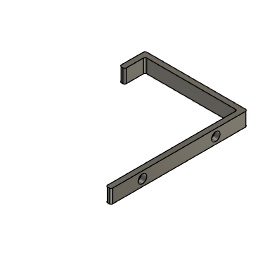
Dell Monitor Mount (Autodesk Fusion 360 design; units mm, degrees)
Autodesk Fusion 360 part; units mm, degrees
sketch "Sketch1" plane through (0, 0, 0) normal (0, 0, 1) x (1, 0, 0)
  line L0 (0, 0) -> (3, 0)
  line L1 (3, 0) -> (3, 80)
  line L2 (3, 80) -> (0, 80)
  line L3 (0, 77) -> (0, 0)
  line L4 (0, 80) -> (-57, 80)
  line L5 (-57, 80) -> (-57, 77)
  line L6 (-54, 77) -> (0, 77)
  line L7 (-54, 77) -> (-54, 65)
  line L8 (-54, 65) -> (-57, 65)
  line L9 (-57, 65) -> (-57, 77)
  dimension "d1" = 80
  dimension "d2" = 3
  dimension "d3" = 60
  dimension "d4" = 3
  dimension "d5" = 15
  dimension "d6" = 3
  constraint horizontal L0
  constraint vertical L1
  constraint horizontal L2
  constraint vertical L3
  constraint coincident L0.start L3.end
  constraint horizontal L4
  constraint vertical L5
  constraint horizontal L6
  constraint vertical L7
  constraint horizontal L8
  constraint vertical L9
  measures "d1" distance of L0.end L1.end
  measures "d2" distance of L0.start L0.end
  measures "d3" distance of L1 L5
  measures "d4" distance of L4 L6
  measures "d5" distance of L4 L8
  measures "d6" distance of L7.end L8.end
extrude "Extrude1" add sketch "Sketch1" along normal blind 8
fillet "Fillet1" radius 1 8 edges at (0, 77, 4) (-54, 77, 4) (-54, 65, 4) (-57, 65, 4) (-57, 80, 4) (3, 80, 4) (3, 0, 4) (0, 0, 4)
sketch "Sketch2" plane through (3, 0, 0) normal (1, 0, 0) x (0, 1, 0)
  line L0 (1, 8) -> (1, 0)
  line L1 (1, 0) -> (79, 0)
  line L2 (79, 0) -> (79, 8)
  line L3 (79, 8) -> (1, 8)
  line L4 (80, 0) -> (80, 8)
  point P0 (61.5, 3.944)
  point P1 (18.5, 3.944)
  dimension "d11" = 43
  dimension "d12" = 18.5
  measures "d11" distance of P0 P1
  measures "d12" distance of P0 L4
hole "Hole1" at (3, 61.5, 3.944) at (3, 18.5, 3.944) direction (-1, 0, 0) diameter 5 depth 3 tip angle 118
equation "d12 = ( ( 80 - 43 ) / 2 ) * 1 mm"
